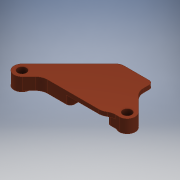
# Autodesk Inventor part: EPS_RegulatorHeatsinkClamp
Saved by Autodesk Inventor 2018 (Build 220112000, 112)
## iProperties
Created: 2020-12-05
Part Number: EPS_RegulatorHeatsinkClamp
Material: Copper
Document SubType Name: Modeling
Designer: Bradley
Mass: 5.75396 g
Surface Area: 7.61096 cm^2
Volume: 0.64362 cm^3
Density: 8.94 g/cm^3
Appearance: Copper - Satin
Author: Bradley
Autodesk Inventor part; units mm, degrees
ref_plane "YZ Plane" through (0, 0, 0) normal (1, 0, 0) x (0, 1, 0)
ref_plane "XZ Plane" through (0, 0, 0) normal (0, 1, 0) x (-1, 0, 0)
ref_plane "XY Plane" through (0, 0, 0) normal (0, 0, 1) x (1, 0, 0)
sketch "Sketch1" plane through (0, 0, 0) normal (0, 0, 1) x (1, 0, 0)
  circle A0 centre (7.3, -3.4) radius 1.1
  circle A1 centre (-15.1, -7.5) radius 1.1
  line L0 (-4.1, 6.3284) -> (4.1, 6.3284)
  line L1 (-4.1, -6.3284) -> (4.1, -6.3284)
  line L2 (0, 6.3284) -> (0, -6.3284) construction
  line L3 (4.1, 6.3284) -> (4.1, -6.3284)
  line L4 (-4.1, 6.3284) -> (-4.1, -6.3284)
  circle A2 centre (7.3, -3.4) radius 2
  circle A3 centre (-15.1, -7.5) radius 2
  line L5 (7.3, -5.4) -> (4.1, -5.4)
  line L6 (8.7142, -1.9858) -> (4.1, 2.6284)
  line L7 (-4.1, -6.3284) -> (-11.1, -6.3284)
  line L8 (-11.1, -6.3284) -> (-13.6858, -8.9142)
  line L9 (-16.5142, -6.0858) -> (-4.1, 6.3284)
  point P0 (0, 0)
  point P1 (0, 0)
  dimension "d0" = 7.3
  dimension "d1" = 3.4
  dimension "d2" = 15.1
  dimension "d3" = 7.5
  dimension "d4" = 2.2
  dimension "d6" = 8.2
  dimension "d7" = 4
  dimension "d8" = 4
  dimension "d9" = 45
  constraints: 20 end point, 4 centre point, 4 point on circle, 4 tangent, 3 coincident, 3 horizontal, 3 midpoint, 3 parallel, 3 perpendicular, 2 point on line, 2 vertical alignment, 1 equal radius, 1 vertical
  measures "d0" horizontal distance of A0.centre point (0, 0)
  measures "d1" vertical distance of point (0, 0) A0.centre
  measures "d2" horizontal distance of A1.centre point (0, 0)
  measures "d3" vertical distance of A1.centre point (0, 0)
  measures "d4" diameter of A1
  measures "d6" distance of L0.start L0.end
  measures "d7" diameter of A2
  measures "d8" diameter of A3
  measures "d9" angle of L5 L6
extrude "Extrusion1" add sketch "Sketch1" along normal blind 3
extrude "Extrusion2" add sketch "Sketch1" against normal blind 0.3 contours A3 | A2
extrude "Extrusion3" cut sketch "Sketch1" along normal blind 2 contours L0 L3 L1 L4
fillet "Fillet1" radius 3 4 edges at (-11.1, -6.3284, 1.5) (4.1, 2.6284, 2.5) (4.1, -5.4, 2.5) (4.1, -6.3284, 2.5)
fillet "Fillet1" radius 1 5 edges at (4.1, -5.4, 1) (4.1, 2.6284, 1) (-4.1, 6.3284, 1) (-4.1, -6.3284, 1) (4.1, 6.3284, 2.5)
fillet "Fillet1" radius 2 1 edges at (-4.1, 6.3284, 2.5)
body "Solid1"
